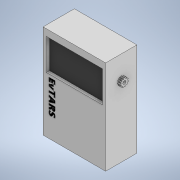
# Autodesk Inventor part: body
Saved by Autodesk Inventor 2021 (Build 250183000, 183)
## iProperties
Created: 2025-04-02
Part Number: body
Material: Generic
Document SubType Name: Modeling
Designer: Admin
Density: 1 g/cm^3
Appearance: Default
Author: Admin
Autodesk Inventor part; units mm, degrees
note: some values were not read from the file. Chosen so that the rebuilt part matches the saved one: direction of "Emboss1".
ref_plane "YZ Plane" through (0, 0, 0) normal (1, 0, 0) x (0, 1, 0)
ref_plane "XZ Plane" through (0, 0, 0) normal (0, 1, 0) x (-1, 0, 0)
ref_plane "XY Plane" through (0, 0, 0) normal (0, 0, 1) x (1, 0, 0)
sketch "Sketch1" plane through (0, 0, 0) normal (0, 1, 0) x (-1, 0, 0)
  line L0 (50, 25) -> (-50, 25)
  line L1 (-50, 25) -> (-50, -25)
  line L2 (-50, -25) -> (50, -25)
  line L3 (50, -25) -> (50, 25)
  line L4 (50, 25) -> (-50, -25) construction
  line L5 (-50, 25) -> (50, -25) construction
  point P0 (0, 0)
  dimension "d0" = 100
  dimension "d1" = 50
  constraints: 12 end point, 2 midpoint, 2 parallel, 1 horizontal, 1 perpendicular
  measures "d0" distance of L2.end L1.end
  measures "d1" distance of L1.end L0.end
extrude "Extrusion1" add sketch "Sketch1" along normal blind 150
sketch "Sketch2" plane through (-50, 0, -25) normal (-1, 0, 0) x (0, 0, 1)
  line L0 (50, 0) -> (50, 150) projected
  line L1 (0, 150) -> (50, 150) projected
  line L2 (25, 119.5) -> (25.5, 119.5)
  line L3 (25.5, 119.5) -> (26.2768, 117.8342)
  line L4 (25, 119.5) -> (24.5, 119.5)
  line L5 (24.5, 119.5) -> (23.7232, 117.8342)
  line L6 (21.4858, 118.4681) -> (21.9065, 118.7385)
  line L7 (21.9065, 118.7385) -> (23.4605, 117.7571)
  line L8 (21.0652, 118.1978) -> (21.3123, 116.3766)
  line L9 (21.4858, 118.4681) -> (21.0652, 118.1978)
  line L10 (19.0874, 115.7002) -> (19.2951, 116.155)
  line L11 (19.2951, 116.155) -> (21.133, 116.1696)
  line L12 (18.8797, 115.2454) -> (20.0722, 113.8468)
  line L13 (19.0874, 115.7002) -> (18.8797, 115.2454)
  line L14 (18.5662, 112.075) -> (18.495, 112.5699)
  line L15 (18.495, 112.5699) -> (20.0333, 113.5758)
  line L16 (18.6373, 111.58) -> (20.3967, 111.0483)
  line L17 (18.5662, 112.075) -> (18.6373, 111.58)
  line L18 (20.0876, 108.7434) -> (19.7602, 109.1213)
  line L19 (19.7602, 109.1213) -> (20.5104, 110.7992)
  line L20 (20.4151, 108.3655) -> (22.1826, 108.8693)
  line L21 (20.0876, 108.7434) -> (20.4151, 108.3655)
  line L22 (23.1687, 106.7633) -> (22.689, 106.9042)
  line L23 (22.689, 106.9042) -> (22.413, 108.7213)
  line L24 (23.6485, 106.6224) -> (24.8631, 108.0019)
  line L25 (23.1687, 106.7633) -> (23.6485, 106.6224)
  line L26 (26.8313, 106.7633) -> (26.3515, 106.6224)
  line L27 (26.3515, 106.6224) -> (25.1369, 108.0019)
  line L28 (27.311, 106.9042) -> (27.587, 108.7213)
  line L29 (26.8313, 106.7633) -> (27.311, 106.9042)
  line L30 (29.9124, 108.7434) -> (29.5849, 108.3655)
  line L31 (29.5849, 108.3655) -> (27.8174, 108.8693)
  line L32 (30.2398, 109.1213) -> (29.4896, 110.7992)
  line L33 (29.9124, 108.7434) -> (30.2398, 109.1213)
  line L34 (31.4338, 112.075) -> (31.3627, 111.58)
  line L35 (31.3627, 111.58) -> (29.6033, 111.0483)
  line L36 (31.505, 112.5699) -> (29.9667, 113.5758)
  line L37 (31.4338, 112.075) -> (31.505, 112.5699)
  line L38 (30.9126, 115.7002) -> (31.1203, 115.2454)
  line L39 (31.1203, 115.2454) -> (29.9278, 113.8468)
  line L40 (30.7049, 116.155) -> (28.867, 116.1696)
  line L41 (30.9126, 115.7002) -> (30.7049, 116.155)
  line L42 (28.5142, 118.4681) -> (28.9348, 118.1978)
  line L43 (28.9348, 118.1978) -> (28.6877, 116.3766)
  line L44 (28.0935, 118.7385) -> (26.5395, 117.7571)
  line L45 (28.5142, 118.4681) -> (28.0935, 118.7385)
  arc A0 (23.7232, 117.8342) -> (23.4605, 117.7571) centre (25, 113) ccw
  arc A1 (26.5395, 117.7571) -> (26.2768, 117.8342) centre (25, 113) ccw
  arc A2 (28.867, 116.1696) -> (28.6877, 116.3766) centre (25, 113) ccw
  arc A3 (29.9667, 113.5758) -> (29.9278, 113.8468) centre (25, 113) ccw
  arc A4 (29.4896, 110.7992) -> (29.6033, 111.0483) centre (25, 113) ccw
  arc A5 (27.587, 108.7213) -> (27.8174, 108.8693) centre (25, 113) ccw
  arc A6 (24.8631, 108.0019) -> (25.1369, 108.0019) centre (25, 113) ccw
  arc A7 (22.1826, 108.8693) -> (22.413, 108.7213) centre (25, 113) ccw
  arc A8 (20.3967, 111.0483) -> (20.5104, 110.7992) centre (25, 113) ccw
  arc A9 (21.3123, 116.3766) -> (21.133, 116.1696) centre (25, 113) ccw
  arc A10 (20.0722, 113.8468) -> (20.0333, 113.5758) centre (25, 113) ccw
  circle A11 centre (25, 113) radius 2.5
  point P0 (25, 0)
  point P1 (25, 118)
  point P2 (22.2968, 117.2063)
  point P3 (20.4518, 115.0771)
  point P4 (20.0509, 112.2884)
  point P5 (21.2213, 109.7257)
  point P6 (23.5913, 108.2025)
  point P7 (26.4087, 108.2025)
  point P8 (28.7787, 109.7257)
  point P9 (29.9491, 112.2884)
  point P10 (29.5482, 115.0771)
  point P11 (27.7032, 117.2063)
  dimension "d5" = 25
  dimension "d6" = 37
  dimension "d8" = 0.5
  dimension "d9" = 115
  dimension "d10" = 6.5
  dimension "d13" = 360
  dimension "d15" = 5
  constraints: 88 end point, 22 point on circle, 12 centre point, 1 coincident, 1 horizontal, 111 other
  measures "d5" distance from line of L0 A0.centre
  measures "d6" distance from line of L1 A0.centre
  measures "d8" distance of L2.start L2.end
  measures "d9" angle of L2 L3
  measures "d10" distance from line of A0.centre L4
  measures "d15" diameter of A11
extrude "Extrusion2" add sketch "Sketch2" along normal blind 5
sketch "Sketch3" plane through (50, 0, 25) normal (1, 0, 0) x (0, 0, -1)
  line L0 (50, 0) -> (50, 150)
  line L1 (0, 150) -> (50, 150)
  line L2 (25, 119.5) -> (25.5, 119.5)
  line L3 (25.5, 119.5) -> (26.2768, 117.8342)
  line L4 (24.5, 119.5) -> (23.7232, 117.8342)
  line L5 (25, 119.5) -> (24.5, 119.5)
  line L6 (21.4858, 118.4681) -> (21.9065, 118.7385)
  line L7 (21.9065, 118.7385) -> (23.4605, 117.7571)
  line L8 (21.0652, 118.1978) -> (21.3123, 116.3766)
  line L9 (21.4858, 118.4681) -> (21.0652, 118.1978)
  line L10 (19.0874, 115.7002) -> (19.2951, 116.155)
  line L11 (19.2951, 116.155) -> (21.133, 116.1696)
  line L12 (18.8797, 115.2454) -> (20.0722, 113.8468)
  line L13 (19.0874, 115.7002) -> (18.8797, 115.2454)
  line L14 (18.5662, 112.075) -> (18.495, 112.5699)
  line L15 (18.495, 112.5699) -> (20.0333, 113.5758)
  line L16 (18.6373, 111.58) -> (20.3967, 111.0483)
  line L17 (18.5662, 112.075) -> (18.6373, 111.58)
  line L18 (20.0876, 108.7434) -> (19.7602, 109.1213)
  line L19 (19.7602, 109.1213) -> (20.5104, 110.7992)
  line L20 (20.4151, 108.3655) -> (22.1826, 108.8693)
  line L21 (20.0876, 108.7434) -> (20.4151, 108.3655)
  line L22 (23.1687, 106.7633) -> (22.689, 106.9042)
  line L23 (22.689, 106.9042) -> (22.413, 108.7213)
  line L24 (23.6485, 106.6224) -> (24.8631, 108.0019)
  line L25 (23.1687, 106.7633) -> (23.6485, 106.6224)
  line L26 (26.8313, 106.7633) -> (26.3515, 106.6224)
  line L27 (26.3515, 106.6224) -> (25.1369, 108.0019)
  line L28 (27.311, 106.9042) -> (27.587, 108.7213)
  line L29 (26.8313, 106.7633) -> (27.311, 106.9042)
  line L30 (29.9124, 108.7434) -> (29.5849, 108.3655)
  line L31 (29.5849, 108.3655) -> (27.8174, 108.8693)
  line L32 (30.2398, 109.1213) -> (29.4896, 110.7992)
  line L33 (29.9124, 108.7434) -> (30.2398, 109.1213)
  line L34 (31.4338, 112.075) -> (31.3627, 111.58)
  line L35 (31.3627, 111.58) -> (29.6033, 111.0483)
  line L36 (31.505, 112.5699) -> (29.9667, 113.5758)
  line L37 (31.4338, 112.075) -> (31.505, 112.5699)
  line L38 (30.9126, 115.7002) -> (31.1203, 115.2454)
  line L39 (31.1203, 115.2454) -> (29.9278, 113.8468)
  line L40 (30.7049, 116.155) -> (28.867, 116.1696)
  line L41 (30.9126, 115.7002) -> (30.7049, 116.155)
  line L42 (28.5142, 118.4681) -> (28.9348, 118.1978)
  line L43 (28.9348, 118.1978) -> (28.6877, 116.3766)
  line L44 (28.0935, 118.7385) -> (26.5395, 117.7571)
  line L45 (28.5142, 118.4681) -> (28.0935, 118.7385)
  arc A0 (23.7232, 117.8342) -> (23.4605, 117.7571) centre (25, 113) ccw
  arc A1 (26.5395, 117.7571) -> (26.2768, 117.8342) centre (25, 113) ccw
  arc A2 (28.867, 116.1696) -> (28.6877, 116.3766) centre (25, 113) ccw
  arc A3 (29.9667, 113.5758) -> (29.9278, 113.8468) centre (25, 113) ccw
  arc A4 (29.4896, 110.7992) -> (29.6033, 111.0483) centre (25, 113) ccw
  arc A5 (27.587, 108.7213) -> (27.8174, 108.8693) centre (25, 113) ccw
  arc A6 (24.8631, 108.0019) -> (25.1369, 108.0019) centre (25, 113) ccw
  arc A7 (22.1826, 108.8693) -> (22.413, 108.7213) centre (25, 113) ccw
  arc A8 (20.3967, 111.0483) -> (20.5104, 110.7992) centre (25, 113) ccw
  arc A9 (21.3123, 116.3766) -> (21.133, 116.1696) centre (25, 113) ccw
  arc A10 (20.0722, 113.8468) -> (20.0333, 113.5758) centre (25, 113) ccw
  circle A11 centre (25, 113) radius 2.5
  point P0 (25, 0)
  point P1 (25, 0)
  point P2 (25, 118)
  point P3 (22.2968, 117.2063)
  point P4 (20.4518, 115.0771)
  point P5 (20.0509, 112.2884)
  point P6 (21.2213, 109.7257)
  point P7 (23.5913, 108.2025)
  point P8 (26.4087, 108.2025)
  point P9 (28.7787, 109.7257)
  point P10 (29.9491, 112.2884)
  point P11 (29.5482, 115.0771)
  point P12 (27.7032, 117.2063)
  dimension "d20" = 25
  dimension "d21" = 37
  dimension "d22" = 0.5
  dimension "d23" = 115
  dimension "d24" = 6.5
  dimension "d25" = 360
  dimension "d26" = 5
  constraints: 92 end point, 22 point on circle, 12 centre point, 1 coincident, 1 horizontal, 111 other
  measures "d20" distance from line of L0 A0.centre
  measures "d21" distance from line of L1 A0.centre
  measures "d22" distance of L2.start L2.end
  measures "d23" angle of L2 L3
  measures "d24" distance from line of A0.centre L5
  measures "d26" diameter of A11
extrude "Extrusion3" add sketch "Sketch3" along normal blind 5
sketch "Sketch4" plane through (-50, 0, 25) normal (0, 0, 1) x (1, 0, 0)
  line L0 (9.3138, 85.067) -> (19.3138, 85.067)
  line L1 (19.3138, 85.067) -> (19.3138, 78.8425)
  line L2 (19.3138, 78.8425) -> (16.9576, 78.8425)
  line L3 (16.9576, 78.8425) -> (16.9576, 82.0521)
  line L4 (16.9576, 82.0521) -> (15.5012, 82.0521)
  line L5 (15.5012, 82.0521) -> (15.5012, 79.0373)
  line L6 (15.5012, 79.0373) -> (13.145, 79.0373)
  line L7 (13.145, 79.0373) -> (13.145, 82.0521)
  line L8 (13.145, 82.0521) -> (11.67, 82.0521)
  line L9 (11.67, 82.0521) -> (11.67, 78.6106)
  line L10 (11.67, 78.6106) -> (9.3138, 78.6106)
  line L11 (9.3138, 78.6106) -> (9.3138, 85.067)
  line L12 (9.3138, 72.2562) -> (9.3138, 75.7813)
  line L13 (9.3138, 75.7813) -> (16.4566, 78.1653)
  line L14 (16.4566, 78.1653) -> (16.4566, 75.067)
  line L15 (16.4566, 75.067) -> (12.5605, 74.195)
  spline S0 degree 2 poles (12.5605, 74.195) (11.6143, 73.9909) (11.1412, 73.9631) knots 0 0 0 1 1 1
  line L16 (11.1412, 73.9631) -> (11.1412, 73.926)
  spline S1 degree 2 poles (11.1412, 73.926) (11.2804, 73.9074) (11.5772, 73.8611) (16.4566, 72.8499) knots 0 0 0 1 2 2 2
  line L17 (16.4566, 72.8499) -> (16.4566, 69.7701)
  line L18 (16.4566, 69.7701) -> (9.3138, 72.2562)
  line L19 (16.9576, 63.7312) -> (9.3138, 63.7312)
  line L20 (9.3138, 63.7312) -> (9.3138, 66.7553)
  line L21 (9.3138, 66.7553) -> (16.9576, 66.7553)
  line L22 (16.9576, 66.7553) -> (16.9576, 69.5568)
  line L23 (16.9576, 69.5568) -> (19.3138, 69.5568)
  line L24 (19.3138, 69.5568) -> (19.3138, 60.9019)
  line L25 (19.3138, 60.9019) -> (16.9576, 60.9019)
  line L26 (16.9576, 60.9019) -> (16.9576, 63.7312)
  line L27 (9.3138, 53.4251) -> (11.1505, 53.8611)
  line L28 (11.1505, 53.8611) -> (11.1505, 56.8481)
  line L29 (11.1505, 56.8481) -> (9.3138, 57.3212)
  line L30 (9.3138, 57.3212) -> (9.3138, 60.5772)
  line L31 (9.3138, 60.5772) -> (19.3138, 57.1356)
  line L32 (19.3138, 57.1356) -> (19.3138, 53.3972)
  line L33 (19.3138, 53.3972) -> (9.3138, 50.1505)
  line L34 (9.3138, 50.1505) -> (9.3138, 53.4251)
  line L35 (17.1338, 55.3175) -> (17.1338, 55.3824)
  spline S2 degree 2 poles (17.1338, 55.3824) (16.9669, 55.4009) (16.1969, 55.5679) (13.2934, 56.3286) knots 0 0 0 1 2 2 2
  line L36 (13.2934, 56.3286) -> (13.2934, 54.4176)
  line L37 (13.2934, 54.4176) -> (16.0114, 55.1134)
  spline S3 degree 2 poles (16.0114, 55.1134) (16.6143, 55.2618) (17.1338, 55.3175) knots 0 0 0 1 1 1
  line L38 (9.3138, 43.7868) -> (11.4659, 44.5382)
  spline S4 degree 2 poles (11.4659, 44.5382) (12.106, 44.7516) (12.8296, 45.4473) (12.8296, 45.8462) knots 0 0 0 1 2 2 2
  line L39 (12.8296, 45.8462) -> (12.8296, 45.9668)
  line L40 (12.8296, 45.9668) -> (9.3138, 45.9668)
  line L41 (9.3138, 45.9668) -> (9.3138, 48.9816)
  line L42 (9.3138, 48.9816) -> (19.3138, 48.9816)
  line L43 (19.3138, 48.9816) -> (19.3138, 44.9742)
  spline S5 degree 2 poles (19.3138, 44.9742) (19.3138, 42.8777) (17.9409, 40.874) (16.568, 40.874) knots 0 0 0 1 2 2 2
  spline S6 degree 2 poles (16.568, 40.874) (15.5383, 40.874) (14.1375, 42.0429) (13.8221, 43.1931) knots 0 0 0 1 2 2 2
  line L44 (13.8221, 43.1931) -> (13.7943, 43.1931)
  spline S7 degree 2 poles (13.7943, 43.1931) (13.5995, 42.5531) (12.7275, 41.7089) (11.8555, 41.375) knots 0 0 0 1 2 2 2
  line L45 (11.8555, 41.375) -> (9.3138, 40.3917)
  line L46 (9.3138, 40.3917) -> (9.3138, 43.7868)
  spline S8 degree 2 poles (16.1412, 44.0744) (16.6422, 44.0744) (17.2266, 44.6867) (17.2266, 45.3453) knots 0 0 0 1 2 2 2
  line L47 (17.2266, 45.3453) -> (17.2266, 45.9668)
  line L48 (17.2266, 45.9668) -> (14.9446, 45.9668)
  line L49 (14.9446, 45.9668) -> (14.9446, 45.4195)
  spline S9 degree 2 poles (14.9446, 45.4195) (14.9446, 44.8165) (15.631, 44.0744) (16.1412, 44.0744) knots 0 0 0 1 2 2 2
  spline S10 degree 2 poles (12.3379, 32.2933) (11.3453, 32.2933) (9.8611, 33.3601) (9.1375, 35.2803) (9.1375, 36.6347) knots 0 0 0 1 2 3 3 3
  spline S11 degree 2 poles (9.1375, 36.6347) (9.1375, 38.2024) (9.6663, 39.5104) knots 0 0 0 1 1 1
  line L50 (9.6663, 39.5104) -> (12.4121, 39.5104)
  spline S12 degree 2 poles (12.4121, 39.5104) (11.9483, 38.8796) (11.3824, 37.3675) (11.3824, 36.7089) knots 0 0 0 1 2 2 2
  spline S13 degree 2 poles (11.3824, 36.7089) (11.3824, 36.2173) (11.7349, 35.67) (12.0782, 35.67) knots 0 0 0 1 2 2 2
  spline S14 degree 2 poles (12.0782, 35.67) (12.3286, 35.67) (12.6904, 35.939) (13.0151, 36.4956) (13.2934, 37.2377) knots 0 0 0 1 2 3 3 3
  spline S15 degree 2 poles (13.2934, 37.2377) (14.221, 39.6495) (16.2897, 39.6495) knots 0 0 0 1 1 1
  spline S16 degree 2 poles (16.2897, 39.6495) (17.7461, 39.6495) (19.4808, 37.4418) (19.4808, 35.5865) knots 0 0 0 1 2 2 2
  spline S17 degree 2 poles (19.4808, 35.5865) (19.4808, 35.067) (19.3973, 34.1857) (19.2674, 33.4714) (19.1004, 32.8221) knots 0 0 0 1 2 3 3 3
  line L51 (19.1004, 32.8221) -> (16.5494, 32.8221)
  spline S18 degree 2 poles (16.5494, 32.8221) (17.2451, 34.0837) (17.2451, 35.3082) knots 0 0 0 1 1 1
  spline S19 degree 2 poles (17.2451, 35.3082) (17.2451, 35.8091) (16.8648, 36.4213) (16.5401, 36.4213) knots 0 0 0 1 2 2 2
  spline S20 degree 2 poles (16.5401, 36.4213) (16.2247, 36.4213) (15.8166, 35.9297) (15.4826, 35.1412) knots 0 0 0 1 2 2 2
  spline S21 degree 2 poles (15.4826, 35.1412) (14.8611, 33.5828) (13.3676, 32.2933) (12.3379, 32.2933) knots 0 0 0 1 2 2 2
  point P0 (50, 0)
  point P1 (14.3092, 59.0512)
  constraints: 1 other
emboss "Emboss1" sketch "Sketch4" operation cut depth 0.5 direction (0, 0, -1)
sketch "Sketch5" plane through (-50, 0, 25) normal (0, 0, 1) x (1, 0, 0)
  line L0 (5, 139.4363) -> (95, 139.4363)
  line L1 (95, 139.4363) -> (95, 89.4363)
  line L2 (95, 89.4363) -> (5, 89.4363)
  line L3 (5, 89.4363) -> (5, 139.4363)
  line L4 (5, 139.4363) -> (95, 89.4363) construction
  line L5 (95, 139.4363) -> (5, 89.4363) construction
  point P0 (50, 0)
  point P1 (50, 114.4363)
  dimension "d31" = 90
  dimension "d32" = 50
  constraints: 12 end point, 2 midpoint, 2 parallel, 1 horizontal, 1 perpendicular
  measures "d31" distance of L1.end L2.end
  measures "d32" distance of L0.end L1.end
extrude "Extrusion4" cut sketch "Sketch5" against normal blind 5
body "Solid1"
